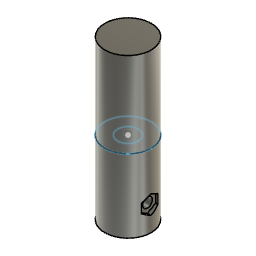
Ruedas (Autodesk Fusion 360 design; units mm, degrees)
Autodesk Fusion 360 part; units mm, degrees
sketch "Boceto1" plane through (0, 0, 0) normal (0, 0, 1) x (1, 0, 0)
  circle A0 centre (0, 30) radius 9.5
  circle A1 centre (0, 30) radius 4.25
  dimension "d12" = 19
  dimension "d32" = 8.5
  constraint concentric A0 A1
  measures "d12" diameter of A0
  measures "d32" diameter of A1
extrude "Extruir2" add sketch "Boceto1" against normal blind 30 makes body 1
extrude "Extruir1" add sketch "Boceto1" along normal blind 35 separate body contours A0 | A1 makes body 2
sketch "Boceto3" plane through (0, 0, 0) normal (0, 1, 0) x (1, 0, 0)
sketch "Boceto4" plane through (0, 0, 0) normal (1, 0, 0) x (0, 1, 0)
  line L0 (30, -30) -> (30, -20)
  circle A0 centre (30, -20) radius 2.9
  line L1 (30, -20) -> (30, -23.1736)
  line L2 (30, -20) -> (30, -23.88)
  line L3 (30, -20) -> (26.61, -20)
  circle A1 centre (30, -20) radius 2
  line L4 (30, -23.88) -> (27.8617, -22.6476)
  line L5 (26.61, -20) -> (26.61, -21.9262)
  line L6 (27.8617, -22.6476) -> (26.61, -21.9262)
  line L7 (26.61, -18.0739) -> (26.61, -20.0001)
  line L8 (30, -23.88) -> (27.8617, -22.6476)
  line L9 (30, -20) -> (30, -16.12)
  line L10 (30, -16.12) -> (26.61, -18.0739)
  line L11 (30, -16.8277) -> (30, -17.1)
  line L12 (30, -18) -> (30, -20.0013)
  line L13 (30, -20.0013) -> (33.39, -20.0013)
  line L14 (33.39, -20.0013) -> (33.39, -18.0739)
  line L15 (33.39, -18.0739) -> (30, -16.12)
  line L16 (33.39, -20.0013) -> (33.39, -21.9262)
  line L17 (33.39, -21.9262) -> (30, -23.88)
  dimension "d13" = 10
  dimension "d14" = 5.8
  dimension "d15" = 3.88
  dimension "d16" = 3.39
  dimension "d17" = 4
  dimension "d18" = 3.88
  dimension "d19" = 3.39
  constraint vertical L0
  constraint coincident L0.end A0.centre
  constraint coincident L0 L1.end
  constraint parallel L0 L1
  constraint parallel L1 L2
  constraint perpendicular L2 L3
  constraint concentric A0 A1
  constraint perpendicular L3 L5
  constraint parallel L4 L6
  constraint parallel L9 L11
  constraint coincident A0 L11.end
  constraint coincident A1 L12.start
  constraint collinear L11 L12
  constraint perpendicular L7 L13
  constraint perpendicular L13 L14
  constraint perpendicular L13 L16
  measures "d13" distance of L0.start L0.end
  measures "d14" diameter of A0
  measures "d15" distance of L0.end L2.end
  measures "d16" distance of L0.end L3.end
  measures "d17" diameter of A1
  measures "d18" distance of L0.end L9.end
  measures "d19" distance of L12.end L13.end
ref_plane "PlanoDeObra1" through (8, 0, 0) normal (1, 0, 0) x (0, 1, 0)
sketch "Boceto5" plane through (8, 0, 0) normal (1, 0, 0) x (0, 1, 0)
  line L0 (30, -16.12) -> (26.61, -18.0739)
  circle A0 centre (30, -20) radius 2
  line L1 (30, -18) -> (30, -20.0013)
  circle A1 centre (30, -20) radius 2.9
  line L2 (30, -20) -> (30, -16.12)
  line L3 (33.39, -20.0013) -> (33.39, -18.0739)
  line L4 (30, -20.0013) -> (33.39, -20.0013)
  line L5 (33.39, -20.0013) -> (33.39, -21.9262)
  line L6 (30, -30) -> (30, -20)
  line L7 (30, -23.88) -> (27.8617, -22.6476)
  line L8 (27.8617, -22.6476) -> (26.61, -21.9262)
  line L9 (30, -23.88) -> (27.8617, -22.6476)
  line L10 (26.61, -20) -> (26.61, -21.9262)
  line L11 (30, -20) -> (26.61, -20)
  line L12 (26.61, -18.0739) -> (26.61, -20.0001)
  line L13 (30, -16.12) -> (33.39, -18.0739)
  line L14 (30, -23.88) -> (33.39, -21.9262)
  point P0 (30, -23.1736)
  point P1 (30, -17.1)
  point P2 (30, -16.8277)
  dimension "d21" = 10
  dimension "d22" = 5.8
  dimension "d23" = 3.39
  dimension "d24" = 4
  dimension "d25" = 3.88
  dimension "d26" = 3.39
  constraint vertical L6
  constraint coincident A0.centre A1.centre
  constraint coincident P0 L6
  constraint concentric A0 A1
  constraint perpendicular L10 L11
  constraint parallel L7 L8
  constraint coincident P1 A1
  constraint coincident L1.start A0
  constraint perpendicular L4 L12
  constraint perpendicular L3 L4
  constraint perpendicular L4 L5
  measures "d21" distance of L6.start A0.centre
  measures "d22" diameter of A1
  measures "d23" distance of L10.start A0.centre
  measures "d24" diameter of A0
  measures "d25" distance of A0.centre L0.start
  measures "d26" distance of L1.end L3.start
extrude "Extruir5" cut sketch "Boceto5" along normal blind 2.5 bodies 1
hole "Agujero1" at (8, 30, -20) direction (-1, 0, 0) diameter 4 depth 30 tip angle 118 bodies 1
